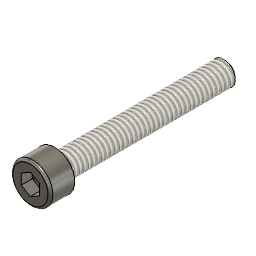
V8 Engine (Autodesk Fusion 360 archive; units mm, degrees)
design "Hexagon Socket Head Cap Screw ASME B18.3 - 5-44 UNF x 7/8 Steel Grade 2 Plain"
description: Hexagon Socket Head Cap Screw ASME B18.3 - 5-44 UNF x 7/8
part number: HSHCS ASME B18.3 - 5-44 UNF x 7/8 Steel Grade 2 Plain
Autodesk Fusion 360 part; units mm, degrees
sketch "Sketch1" plane through (0, 0, 0) normal (0, 1, 0) x (1, 0, 0)
  line L0 (-1.5875, 0) -> (-1.5875, 22.225)
  line L1 (-1.5875, 22.225) -> (0, 22.225)
  line L2 (0, 22.225) -> (0, -3.175)
  line L3 (-1.5875, 0) -> (-2.6035, 0)
  line L4 (-2.6035, 0) -> (-2.6035, -3.175)
  line L5 (-2.6035, -3.175) -> (0, -3.175)
  dimension "d107" = 3.175
  dimension "d108" = 22.225
  dimension "d114" = 5.207
  dimension "d115" = 3.175
  constraint perpendicular L0 L1
  constraint collinear origin L1.end L2.end
  constraint perpendicular L0 L3
  constraint coincident origin L3
  constraint vertical L2
  constraint coincident L2 L5.end
  constraint perpendicular L2 L5
  measures "d107" distance of L3.end L5
  measures "d108" distance of origin L1
revolve "Revolve1" add sketch "Sketch1" angle 360 about axis through (0, 0, -22.225) along (0, 0, 1)
ref_plane "WorkPlane1" through (0, 0, 3.175) normal (0, 0, 1) x (1, 0, 0)
sketch "Sketch6" plane through (0, 0, 3.175) normal (0, 0, 1) x (1, 0, 0)
  line L0 (-1.1938, 0.6892) -> (-1.1938, -0.6892)
  line L1 (-1.1938, -0.6892) -> (0, -1.3785)
  line L2 (0, -1.3785) -> (1.1938, -0.6892)
  line L3 (1.1938, -0.6892) -> (1.1938, 0.6892)
  line L4 (1.1938, 0.6892) -> (0, 1.3785)
  line L5 (0, 1.3785) -> (-1.1938, 0.6892)
  dimension "d116" = 2.3876
  constraint vertical L3
  measures "d116" distance of L0 L3
extrude "Extrude1" cut sketch "Sketch6" against normal blind 1.4478
extrude "Extrude2" cut 1 faces at (-0.3979, -0.2297, 1.7272) along direction (0, 0, -1) blind 1.4478 draft -85
thread "Thread3" "ANSI Unified Screw Threads 0.125(#5) 5-44 UNF 5-44 UNF 2A" major diameter 3.0963 minor diameter 2.4689 pitch 0.5773 angle 60 resizes the face on face at (-1.5855, 0.0791, -14.8167) from (0, 0, -0.8661) to (0, 0, -22.225)
fillet "Fillet4" radius 0.3175 1 edges at (-2.4273, 0.9415, 3.175)
sketch "Sketch7" plane through (0, 0, 0) normal (0, 1, 0) x (1, 0, 0)
  line L0 (-1.6193, 22.225) -> (-1.6193, 21.8808)
  line L1 (-1.6193, 21.8808) -> (-1.2433, 22.225)
  line L2 (0, 22.225) -> (0, -3.175)
  line L3 (-1.6193, 22.225) -> (0, 22.225)
  dimension "d103" = 1.6193
  dimension "d110" = 1.2433
  dimension "d111" = 0.3442
  constraint coincident L2.start L3.end
  constraint perpendicular L2 L3
  constraint coincident L1.end L3
  constraint perpendicular L0 L3
  measures "d103" distance of origin L0
  measures "d110" distance of L1.end L2
  measures "d111" distance of L0.end L3
revolve "Revolve3" cut sketch "Sketch7" angle 360 about axis through (0, 0, 1.75) along (0, 0, 1)
equation "d31 = -adsk_phildepth"
equation "d71 = adsk_headh"
equation "d76 = -adsk_phildepth"
equation "adsk_nomlen = 0.875 in"
equation "adsk_headh = 0.125 in"
equation "adsk_headdia = 0.205 in"
equation "adsk_nomdia = 0.125 in"
equation "adsk_philwidth = 0.094 in"
equation "adsk_phildepth = 0.057 in"
equation "adsk_thrlen = 0.8409021 in"
equation "d93 = adsk_nomdia * 0.1"
equation "adsk_startlen = 0.01355 in"
equation "adsk_endpointdia = 0.0979 in"
equation "d103 = adsk_nomdia * 0.51"
equation "d107 = adsk_headh"
equation "d108 = adsk_nomlen"
equation "d110 = adsk_endpointdia / 2"
equation "d111 = adsk_startlen"
equation "d113 = min(adsk_thrlen; adsk_nomlen - 0.001 mm)"
equation "d114 = adsk_headdia"
equation "d115 = adsk_nomdia"
equation "d116 = adsk_philwidth"
